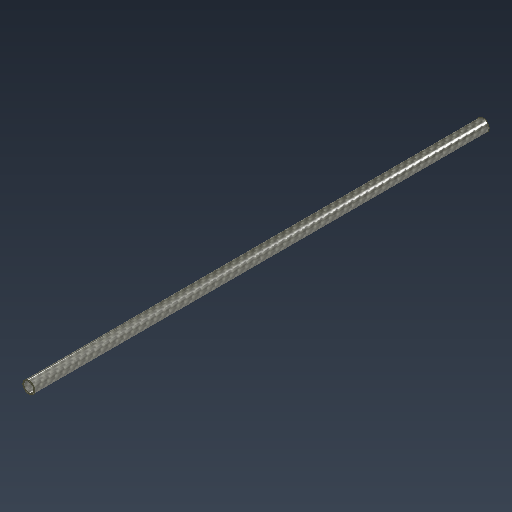
# Autodesk Inventor part: Tube_12x1x_<LoadpipeLength>_CFRP
Saved by Autodesk Inventor 2025 (Build 290162010, 162A)
## iProperties
Created: 2023-06-08
Part Number: Tube_12x1x_<LoadpipeLength>_CFRP
Material: CFRP
Document SubType Name: Modeling
Designer: dzw04
Density: 1.43 g/cm^3
Appearance: Carbon Fiber 1
Mass: 22.2378 g
Surface Area: 311.709 cm^2
Volume: 15.5509 cm^3
Author: dzw04
Autodesk Inventor part; units mm, degrees
ref_plane "YZ Plane" through (0, 0, 0) normal (1, 0, 0) x (0, 1, 0)
ref_plane "XZ Plane" through (0, 0, 0) normal (0, 1, 0) x (-1, 0, 0)
ref_plane "XY Plane" through (0, 0, 0) normal (0, 0, 1) x (1, 0, 0)
sketch "Sketch1" plane through (0, 0, 0) normal (0, 0, 1) x (1, 0, 0)
  circle A0 centre (0, 0) radius 6
  circle A1 centre (0, 0) radius 5
  dimension "d0" = 12
  dimension "d1" = 10
  constraints: 2 centre point, 2 coincident
  measures "d0" diameter of A0
  measures "d1" diameter of A1
extrude "Extrusion1" add sketch "Sketch1" along normal blind 450
equation "\"d2\" = LoadpipeLength"
equation "\"MountToMotorCenter\" = 0"
equation "\"ArmPosition\" = 5deg"
equation "\"LoadpipeLength\" = 450"
equation "\"BatteryWidth\" = 62"
equation "\"BatteryHeight\" = 76"
equation "\"ThicknessBodyOuterPlate\" = 2"
equation "\"ThicknessBodyCenterPlate\" = 2"
equation "\"ThicknessLegLoadpipePlate\" = 2"
equation "\"ThicknessBatteryTray\" = 2"
equation "\"ThicknessBatteryTopTray\" = 1"
equation "\"LandingGearStabilityBar\" = 525"
equation "\"StartAngleArm\" = 45deg"
equation "\"MotorMountCenter\" = 71.5"
body "Solid1"
